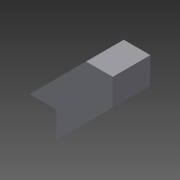
# Autodesk Inventor part: end
Saved by Autodesk Inventor 2015 (Build 190159000, 159)
## iProperties
Created: 2019-04-11
Part Number: end
Material: Generic
Document SubType Name: Modeling
Designer: Raptor
Density: 1 g/cm^3
Appearance: Default
Author: Raptor
Autodesk Inventor part; units mm, degrees
ref_plane "YZ Plane" through (0, 0, 0) normal (1, 0, 0) x (0, 1, 0)
ref_plane "XZ Plane" through (0, 0, 0) normal (0, 1, 0) x (-1, 0, 0)
ref_plane "XY Plane" through (0, 0, 0) normal (0, 0, 1) x (1, 0, 0)
sketch "Sketch1" plane through (0, 0, 0) normal (0, 1, 0) x (-1, 0, 0)
  line L0 (0, 0) -> (0, -70.7107)
  line L1 (70.7107, 0) -> (0, 0)
  line L2 (0, -70.7107) -> (150, -220.7107)
  line L3 (150, -220.7107) -> (150, -150)
  line L4 (150, -150) -> (220.7107, -150)
  line L5 (220.7107, -150) -> (70.7107, 0)
  dimension "d8" = 45
  dimension "d9" = 100
  dimension "d14" = 150
  constraints: 12 end point, 2 equal length, 2 perpendicular, 2 vertical, 1 parallel
  measures "d8" angle of L2 L0
  measures "d9" distance between parallel lines of L2 L5
  measures "d14" distance between parallel lines of L3 L0
extrude "Extrusion1" add sketch "Sketch1" along normal blind 100
body "Solid1"
